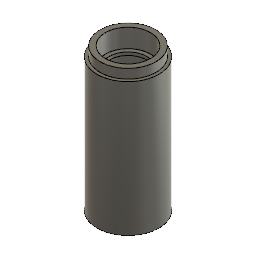
microphone_tube v1 (Autodesk Fusion 360 design; units mm, degrees)
Autodesk Fusion 360 part; units mm, degrees
sketch "Sketch1" plane through (0, 0, 0) normal (0, 1, 0) x (1, 0, 0)
  circle A0 centre (0, 0) radius 10
  dimension "d1" = 20
  measures "d1" diameter of A0
extrude "Extrude1" add sketch "Sketch1" along normal blind 46
sketch "Sketch2" plane through (0, 0, 0) normal (0, 1, 0) x (1, 0, 0)
  circle A0 centre (0, 0) radius 8
  dimension "d4" = 16
  measures "d4" diameter of A0
extrude "Extrude2" cut sketch "Sketch2" along normal blind 39
sketch "Sketch3" plane through (0, 46, 0) normal (0, 1, 0) x (-1, 0, 0)
  circle A0 centre (0, 0) radius 10
  circle A1 centre (0, 0) radius 9
  dimension "d7" = 18
  measures "d7" diameter of A1
extrude "Extrude3" cut sketch "Sketch3" against normal blind 3
sketch "Sketch4" plane through (0, 46, 0) normal (0, 1, 0) x (-1, 0, 0)
  circle A0 centre (0, 0) radius 9
  circle A1 centre (0, 0) radius 7.265
  dimension "d10" = 14.53
  measures "d10" diameter of A1
extrude "Extrude4" cut sketch "Sketch4" against normal blind 6 contours A1
sketch "Sketch5" plane through (0, 40, 0) normal (0, 1, 0) x (-1, 0, 0)
  circle A0 centre (0, 0) radius 7.265
  circle A1 centre (0, 0) radius 6
  dimension "d13" = 12
  measures "d13" diameter of A1
extrude "Extrude5" cut sketch "Sketch5" against normal blind 10 contours A1
